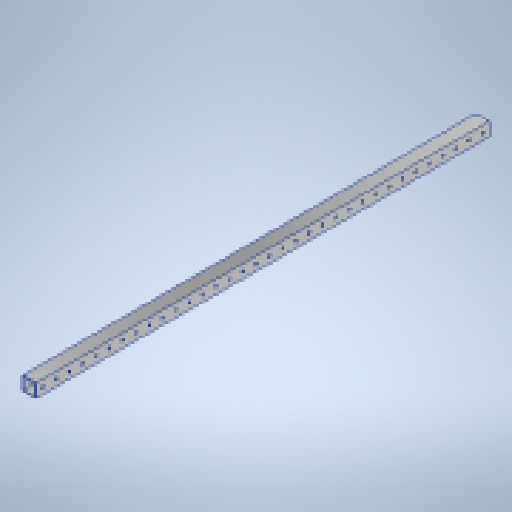
# Autodesk Inventor part: Angled_bar
Saved by Autodesk Inventor 2024 (Build 280153000, 153)
## iProperties
Created: 2023-04-21
Part Number: Angled_bar
Material: Aluminum 6061
Document SubType Name: Modeling
Designer: legom
Density: 2.7 g/cm^3
Appearance: Aluminum - Flat
Author: legom
Autodesk Inventor part; units mm, degrees
ref_plane "YZ Plane" through (0, 0, 0) normal (1, 0, 0) x (0, 1, 0)
ref_plane "XZ Plane" through (0, 0, 0) normal (0, 1, 0) x (-1, 0, 0)
ref_plane "XY Plane" through (0, 0, 0) normal (0, 0, 1) x (1, 0, 0)
sketch "Sketch1" plane through (0, 0, 0) normal (0, 0, 1) x (1, 0, 0)
  line L0 (0, 0) -> (25.4, 0)
  line L1 (25.4, 0) -> (25.4, 25.4)
  line L2 (25.4, 25.4) -> (0, 25.4)
  line L3 (0, 25.4) -> (0, 0)
  line L4 (23.114, 2.286) -> (2.286, 2.286)
  line L5 (2.286, 2.286) -> (2.286, 23.114)
  line L6 (2.286, 23.114) -> (23.114, 23.114)
  line L7 (23.114, 23.114) -> (23.114, 2.286)
  dimension "d0" = 25.4
  dimension "d1" = 25.4
  dimension "d2" = 2.286
  constraints: 16 end point, 4 parallel, 2 perpendicular, 1 horizontal, 3 other
  measures "d0" distance of L2.end L1.end
  measures "d1" distance of L1.end L0.end
  measures "d2" distance between parallel lines of L0 L4
extrude "Extrusion1" add sketch "Sketch1" along normal blind 863.6
sketch "Sketch2" plane through (25.4, 0, 0) normal (1, 0, 0) x (0, 0, -1)
  circle A0 centre (-12.7, 12.7) radius 2.5527
  line L0 (0, 25.4) -> (-863.6, 25.4) projected
  line L1 (0, 0) -> (0, 25.4) projected
  circle A1 centre (-38.1, 12.7) radius 2.5527
  circle A2 centre (-63.5, 12.7) radius 2.5527
  circle A3 centre (-88.9, 12.7) radius 2.5527
  circle A4 centre (-114.3, 12.7) radius 2.5527
  circle A5 centre (-139.7, 12.7) radius 2.5527
  circle A6 centre (-165.1, 12.7) radius 2.5527
  circle A7 centre (-190.5, 12.7) radius 2.5527
  circle A8 centre (-215.9, 12.7) radius 2.5527
  circle A9 centre (-241.3, 12.7) radius 2.5527
  circle A10 centre (-266.7, 12.7) radius 2.5527
  circle A11 centre (-292.1, 12.7) radius 2.5527
  circle A12 centre (-317.5, 12.7) radius 2.5527
  circle A13 centre (-342.9, 12.7) radius 2.5527
  circle A14 centre (-368.3, 12.7) radius 2.5527
  circle A15 centre (-393.7, 12.7) radius 2.5527
  circle A16 centre (-419.1, 12.7) radius 2.5527
  circle A17 centre (-444.5, 12.7) radius 2.5527
  circle A18 centre (-469.9, 12.7) radius 2.5527
  circle A19 centre (-495.3, 12.7) radius 2.5527
  circle A20 centre (-520.7, 12.7) radius 2.5527
  circle A21 centre (-546.1, 12.7) radius 2.5527
  circle A22 centre (-571.5, 12.7) radius 2.5527
  circle A23 centre (-596.9, 12.7) radius 2.5527
  circle A24 centre (-622.3, 12.7) radius 2.5527
  circle A25 centre (-647.7, 12.7) radius 2.5527
  circle A26 centre (-673.1, 12.7) radius 2.5527
  circle A27 centre (-698.5, 12.7) radius 2.5527
  circle A28 centre (-723.9, 12.7) radius 2.5527
  circle A29 centre (-749.3, 12.7) radius 2.5527
  circle A30 centre (-774.7, 12.7) radius 2.5527
  circle A31 centre (-800.1, 12.7) radius 2.5527
  circle A32 centre (-825.5, 12.7) radius 2.5527
  circle A33 centre (-850.9, 12.7) radius 2.5527
  point P0 (0, 12.7)
  dimension "d5" = 5.1054
  dimension "d6" = 12.7
  dimension "d7" = 12.7
  dimension "d10" = 25.4
  constraints: 34 centre point, 1 horizontal, 1 midpoint, 66 other
  measures "d5" diameter of A0
  measures "d6" distance from line of L0 A0.centre
  measures "d7" distance of A0.centre point (0, 12.7)
  measures "d10" distance of A0.centre A1.centre
extrude "Extrusion2" cut sketch "Sketch2" against normal through all
body "Solid1"
